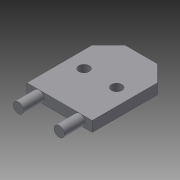
# Autodesk Inventor part: Effector_ZProbe_A
Saved by Autodesk Inventor 2014 (Build 180170000, 170)
## iProperties
Created: 2014-08-28
Part Number: Effector_ZProbe_A
Material: Generic
Document SubType Name: Modeling
Designer: ThatOtherGuy
Density: 1 g/cm^3
Appearance: Default
Author: ThatOtherGuy
Autodesk Inventor part; units mm, degrees
ref_plane "YZ Plane" through (0, 0, 0) normal (1, 0, 0) x (0, 1, 0)
ref_plane "XZ Plane" through (0, 0, 0) normal (0, 1, 0) x (-1, 0, 0)
ref_plane "XY Plane" through (0, 0, 0) normal (0, 0, 1) x (1, 0, 0)
sketch "Sketch1" plane through (0, 0, 0) normal (0, 0, 1) x (1, 0, 0)
  line L0 (0, 0) -> (20, 0)
  line L1 (20, 0) -> (20, 20)
  line L2 (15, 25) -> (5, 25)
  line L3 (0, 20) -> (0, 0)
  circle A0 centre (5, 12.5) radius 1.6
  circle A1 centre (15, 12.5) radius 1.6
  line L4 (5, 25) -> (0, 20)
  line L5 (15, 25) -> (20, 20)
  line L6 (2.1625, 0) -> (2.1625, -6.35)
  line L7 (2.1625, -6.35) -> (5.3375, -6.35)
  line L8 (5.3375, -6.35) -> (5.3375, 0)
  line L9 (14.6625, 0) -> (14.6625, -6.35)
  line L10 (14.6625, -6.35) -> (17.8375, -6.35)
  line L11 (17.8375, -6.35) -> (17.8375, 0)
  point P0 (20, 25)
  point P1 (0, 25)
  dimension "d0" = 25
  dimension "d1" = 20
  dimension "d2" = 3.2
  dimension "d3" = 5
  dimension "d4" = 12.5
  dimension "d7" = 5
  dimension "d8" = 12.5
  dimension "d9" = 5
  dimension "d10" = 5
  dimension "d11" = 5
  dimension "d12" = 5
  dimension "d13" = 3.175
  dimension "d14" = 6.35
  dimension "d15" = 9.325
  dimension "d16" = 2.1625
  dimension "d17" = 2.1625
  constraints: 24 end point, 8 point on line, 5 parallel, 4 perpendicular, 2 centre point, 2 equal length, 1 equal radius, 1 horizontal
  measures "d0" distance of point (0, 25) L0.start
  measures "d1" distance of point (20, 25) point (0, 25)
  measures "d2" diameter of A0
  measures "d3" distance from line of L3 A0.centre
  measures "d4" distance from line of L2 A0.centre
  measures "d7" distance from line of L1 A1.centre
  measures "d8" distance from line of L2 A1.centre
  measures "d9" distance of L2.end point (0, 25)
  measures "d10" distance of L3.start point (0, 25)
  measures "d11" distance of L2.start point (20, 25)
  measures "d12" distance of L1.end point (20, 25)
  measures "d13" distance of L9.end L10.end
  measures "d14" distance of L7.end L8.end
  measures "d15" distance between parallel lines of L9 L8
  measures "d16" distance between parallel lines of L3 L6
  measures "d17" distance between parallel lines of L1 L11
extrude "Extrusion1" add sketch "Sketch1" along normal blind 3.175
sketch "Sketch2" plane through (14.6625, -6.35, 0) normal (0, -1, 0) x (1, 0, 0)
  line L0 (0, 0) -> (3.175, 0) projected
  line L1 (3.175, 0) -> (3.175, 3.175) projected
  line L2 (0, 3.175) -> (3.175, 3.175) projected
  line L3 (0, 0) -> (0, 3.175) projected
  circle A0 centre (1.5875, 1.5875) radius 1.5875
  point P0 (-14.6625, 0)
  constraints: 1 centre point, 1 tangent
extrude "Extrusion2" cut sketch "Sketch2" against normal blind 6.35 contours L3 A0 L0 | A0 L1 L0 | L3 L2 A0 | A0 L2 L1
sketch "Sketch3" plane through (2.1625, -6.35, 0) normal (0, -1, 0) x (1, 0, 0)
  line L0 (0, 0) -> (3.175, 0) projected
  line L1 (3.175, 0) -> (3.175, 3.175) projected
  line L2 (0, 3.175) -> (3.175, 3.175) projected
  line L3 (0, 0) -> (0, 3.175) projected
  circle A0 centre (1.5875, 1.5875) radius 1.5875
  point P0 (-2.1625, 0)
  constraints: 1 centre point, 1 tangent
extrude "Extrusion3" cut sketch "Sketch3" against normal blind 6.35 contours L3 A0 L0 | A0 L1 L0 | L3 L2 A0 | A0 L2 L1
equation "\"d7\" = d3"
equation "\"d8\" = d4"
equation "\"d10\" = d9"
equation "\"d11\" = d9"
equation "\"d12\" = d11"
equation "\"d16\" = d17"
body "Solid1"
